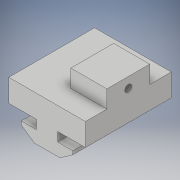
# Autodesk Inventor part: Sliderfor2020
Saved by Autodesk Inventor 2017 (Build 210142000, 142)
## iProperties
Created: 2017-12-08
Part Number: Sliderfor2020
Material: Generic
Document SubType Name: Modeling
Designer: User
Density: 1 g/cm^3
Appearance: Default
Author: User
Autodesk Inventor part; units mm, degrees
ref_plane "YZ Plane" through (0, 0, 0) normal (1, 0, 0) x (0, 1, 0)
ref_plane "XZ Plane" through (0, 0, 0) normal (0, 1, 0) x (-1, 0, 0)
ref_plane "XY Plane" through (0, 0, 0) normal (0, 0, 1) x (1, 0, 0)
sketch "Sketch1" plane through (0, 0, 0) normal (0, 0, 1) x (1, 0, 0)
  line L0 (0, 0) -> (14.5304, 0)
  line L1 (-8.7854, 6.6412) -> (8.2146, 6.6412)
  line L2 (8.2146, 1.6412) -> (2.0946, 1.6412)
  line L3 (2.0946, 1.6412) -> (2.0946, -0.3588)
  line L4 (2.0946, -0.3588) -> (5.4596, -0.3588)
  line L5 (2.5721, -3.1588) -> (-3.1429, -3.1588)
  line L6 (-3.1429, -3.1588) -> (-6.0304, -1.1208)
  line L7 (-6.0304, -1.1208) -> (-6.0304, -0.3588)
  line L8 (-6.0304, -0.3588) -> (-2.6654, -0.3588)
  line L9 (-2.6654, -0.3588) -> (-2.6654, 1.6412)
  line L10 (-2.6654, 1.6412) -> (-8.7854, 1.6412)
  line L11 (-8.7854, 1.6412) -> (-8.7854, 6.6412)
  line L12 (5.4596, -0.3588) -> (5.4596, -1.1208)
  line L13 (5.4596, -1.1208) -> (2.5721, -3.1588)
  line L14 (8.2146, 6.6412) -> (4.8496, 6.6412)
  line L15 (4.8496, 1.6412) -> (8.2146, 1.6412)
  line L16 (8.2146, 6.6412) -> (8.2146, 1.6412)
  dimension "d2" = 5
  dimension "d3" = 2
  dimension "d4" = 4.76
  dimension "d6" = 11.49
  dimension "d7" = 2.755
  dimension "d8" = 5.715
  dimension "d9" = 5.6425
  dimension "d10" = 6.12
  dimension "d11" = 0.762
  dimension "d12" = 0.762
  constraints: 34 end point, 5 perpendicular, 4 point on line, 3 horizontal, 2 vertical, 1 collinear
  measures "d2" distance between parallel lines of L10 L1
  measures "d3" distance between parallel lines of L8 L10
  measures "d4" distance between parallel lines of L3 L9
  measures "d6" distance between parallel lines of L7 L12
  measures "d7" distance between parallel lines of L7 L11
  measures "d8" distance of L5.start L5.end
  measures "d9" distance from line of L5.end L11
  measures "d10" distance between parallel lines of L11 L9
  measures "d11" distance of L6.end L7.end
  measures "d12" distance of L4.end L12.end
extrude "Extrusion1" add sketch "Sketch1" along normal blind 19.05
sketch "Sketch4" plane through (8.2146, 1.6412, 0) normal (1, 0, 0) x (0, 0, -1)
  line L0 (0, 5) -> (0, 0) projected
  line L1 (0, 5) -> (-19.05, 5) projected
  line L2 (-19.05, 0) -> (-19.05, 5) projected
  line L3 (0, 0) -> (-19.05, 0) projected
  line L4 (-9.525, 0) -> (-19.05, 0)
  line L5 (0, 0) -> (-19.05, 0) projected
  line L6 (-4.7625, 0) -> (-14.2875, 0)
  line L7 (-14.2875, 0) -> (-14.2875, 8.89)
  line L8 (-14.2875, 8.89) -> (-4.7625, 8.89)
  line L9 (-4.7625, 8.89) -> (-4.7625, 0)
  point P0 (0, -1.6412)
  dimension "d40" = 19.05
  dimension "d41" = 9.525
  dimension "d42" = 8.89
  dimension "d43" = 4.7625
  constraints: 10 end point, 2 horizontal, 2 parallel, 1 midpoint, 1 perpendicular, 1 point on line
  measures "d40" distance of L0.start L1.end
  measures "d41" distance of L7.end L8.end
  measures "d42" distance of L6.end L7.end
  measures "d43" distance between parallel lines of L0 L9
extrude "Extrusion3" add sketch "Sketch4" against normal blind 8 contours L9 L3 L7 L1 | L1 L7 L8 L9
sketch "Sketch6" plane through (8.2146, 1.6412, 0) normal (1, 0, 0) x (0, 0, -1)
  line L0 (0, 0) -> (-19.05, 0) projected
  line L1 (-4.7625, 8.89) -> (-14.2875, 8.89) projected
  line L2 (-19.05, 0) -> (-19.05, 5) projected
  line L3 (0, 5) -> (0, 0) projected
  circle A0 centre (-9.525, 6.604) radius 1.5
  point P0 (0, -1.6412)
  dimension "d46" = 8.89
  dimension "d47" = 19.05
  dimension "d50" = 3
  dimension "d58" = 6.604
  dimension "d59" = 9.525
  constraints: 1 centre point, 1 coincident
  measures "d46" distance between parallel lines of L0 L1
  measures "d47" distance between parallel lines of L2 L3
  measures "d50" diameter of A0
  measures "d58" distance from line of L0 A0.centre
  measures "d59" distance from line of L2 A0.centre
hole "Hole2" at (8.2146, 8.2452, 9.525) direction (-1, 0, 0) diameter 1.5748 end through all
equation "\"d7\" = -0.5 * d6 + 0.5 * d0"
equation "\"d9\" = -0.5 * d8 + 0.5 * d0"
equation "\"d10\" = -0.5 * d4 + 0.5 * d0"
equation "\"d12\" = d11"
equation "\"d43\" = -0.5 * d41 + 0.5 * d40"
equation "\"d59\" = 0.5 * d47"
equation "\"d0\" = 17"
body "Solid1"
